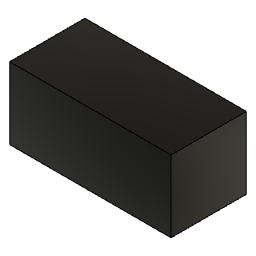
Hippo-PD Test Jig (Autodesk Fusion 360 archive; units mm, degrees)
design "5A regulator"
Autodesk Fusion 360 part; units mm, degrees
sketch "Sketch1" plane through (0, 0, 0) normal (0, 0, 1) x (1, 0, 0) in component "5A regulator"
  line L0 (-22.5, 10.5) -> (22.5, 10.5)
  line L1 (22.5, 10.5) -> (22.5, -10.5)
  line L2 (22.5, -10.5) -> (-22.5, -10.5)
  line L3 (-22.5, -10.5) -> (-22.5, 10.5)
  line L4 (0, 10.5) -> (0, -10.5) construction
  line L5 (-22.5, 0) -> (22.5, 0) construction
  dimension "d5_1" = 21
  dimension "d6_1" = 45
  constraint horizontal L0
  constraint vertical L1
  constraint horizontal L2
  constraint vertical L3
  constraint midpoint L0 L4.start
  constraint midpoint L2 L4.end
  constraint midpoint L3 L5.start
  constraint midpoint L1 L5.end
  constraint coincident origin L5
  constraint coincident origin L4
  measures "d5_1" vertical distance of L0.end L1.end
  measures "d6_1" horizontal distance of L1.end L2.end
extrude "Extrude1" add sketch "Sketch1" along normal blind 20 in component "5A regulator"
component "5A regulator" placed x (1, 0, 0) y (0, 1, 0) z (0, 0, 1) at (0, 0, 0)
